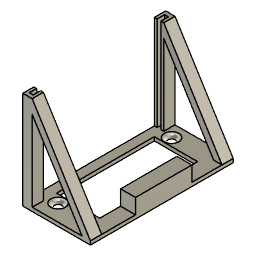
Light Mount Bracket (Autodesk Fusion 360 design; units mm, degrees)
Autodesk Fusion 360 part; units mm, degrees
sketch "Sketch1" plane through (0, 0, 0) normal (0, 0, 1) x (1, 0, 0)
  line L0 (-5, 11) -> (31, 11)
  line L1 (31, 11) -> (31, -65)
  line L2 (31, -65) -> (-5, -65)
  line L3 (-5, -65) -> (-5, 11)
  line L4 (0, 0) -> (23, 0)
  line L5 (23, 0) -> (23, -52)
  line L6 (23, -52) -> (0, -52)
  line L7 (0, -52) -> (0, 0)
  circle A0 centre (5, -56.1622) radius 1.9
  circle A1 centre (5, 4.1628) radius 1.9
  dimension "d1" = 76
  dimension "d2" = 36
  dimension "d3" = 23
  dimension "d4" = 3.8
  dimension "d5" = 60.325
  dimension "d8" = 10
  dimension "d19" = 5
  dimension "d20" = 10
  dimension "d21" = 4.1622
  dimension "d22" = 13
  constraint horizontal L0
  constraint vertical L1
  constraint horizontal L2
  constraint vertical L3
  constraint horizontal L4
  constraint vertical L5
  constraint horizontal L6
  constraint vertical L7
  constraint coincident L4.start L7.end
  constraint equal A0 A1
  measures "d1" distance of L0.start L2.end
  measures "d2" distance of L0.start L0.end
  measures "d3" distance of L4.start L4.end
  measures "d4" diameter of A0
  measures "d5" distance of A0.centre A1.centre
  measures "d8" distance of L3 A0.centre
  measures "d19" distance of L3 L7
  measures "d20" distance of L3 A1.centre
  measures "d21" distance of L6 A0.centre
  measures "d22" distance of L2 L6
extrude "Extrude1" add sketch "Sketch1" along normal blind 2
fillet "Fillet1" radius 2 2 edges at (3.2286, 4.8499, 2) (3.2286, -55.4751, 2)
sketch "Sketch2" plane through (0, 0, 2) normal (0, 0, 1) x (-1, 0, 0)
  circle A0 centre (-5, -4.1628) radius 3.9
  line L0 (-23, 52) -> (0, 52)
  line L1 (0, 52) -> (0, 0)
  line L2 (0, 0) -> (-23, 0)
  line L3 (-23, 0) -> (-23, 52)
  line L4 (5, 65) -> (-31, 65)
  line L5 (-31, 65) -> (-31, -11)
  line L6 (-31, -11) -> (5, -11)
  line L7 (5, -11) -> (5, 65)
  circle A1 centre (-5, 56.1622) radius 3.9
  line L8 (-23, 11) -> (-31, 11)
  line L9 (-31, 11) -> (-31, 41)
  line L10 (-31, 41) -> (-23, 41)
  line L11 (-23, 41) -> (-23, 11)
  dimension "d17" = 30
  dimension "d18" = 22
  constraint horizontal L8
  constraint vertical L9
  constraint horizontal L10
  constraint vertical L11
  constraint coincident L5 L9.end
  constraint collinear L3 L11
  measures "d17" distance of L8 L10
  measures "d18" distance of L6 L8
extrude "Extrude2" add sketch "Sketch2" along normal blind 8 contours L3 L5 L8 L9 L10 L11
sketch "Sketch3" plane through (23, 0, 0) normal (-1, 0, 0) x (0, -1, 0)
  line L0 (0, 0) -> (52, 0)
  line L1 (52, 0) -> (52, 2)
  line L2 (0, 2) -> (0, 0)
  circle A0 centre (26, 7.5) radius 0.625
  line L3 (52, 2) -> (41, 2)
  line L4 (11, 2) -> (0, 2)
  line L5 (41, 2) -> (41, 10)
  line L6 (41, 10) -> (11, 10)
  line L7 (11, 10) -> (11, 2)
  dimension "d16" = 1.25
  dimension "d37" = 2.5
  dimension "d38" = 15
  measures "d16" diameter of A0
  measures "d37" distance of A0.centre L6
  measures "d38" distance of A0.centre L7
extrude "Extrude3" cut sketch "Sketch3" against normal blind 5 contours A0
sketch "Sketch4" plane through (0, 0, 2) normal (0, 0, 1) x (-1, 0, 0)
  line L0 (-23, 11) -> (-31, 11)
  line L1 (-31, 11) -> (-31, -11)
  line L2 (-31, -11) -> (5, -11)
  line L3 (5, -11) -> (5, 65)
  line L4 (5, 65) -> (-31, 65)
  line L5 (-31, 65) -> (-31, 41)
  line L6 (-31, 41) -> (-23, 41)
  line L7 (-23, 41) -> (-23, 52)
  line L8 (-23, 52) -> (0, 52)
  line L9 (0, 52) -> (0, 0)
  line L10 (0, 0) -> (-23, 0)
  line L11 (-23, 0) -> (-23, 11)
  circle A0 centre (-5, -4.1628) radius 3.9
  circle A1 centre (-5, 56.1622) radius 3.9
  line L12 (5, -11) -> (-0.033, -11)
  line L13 (-0.033, -11) -> (-0.033, 65)
  line L14 (-0.033, 65) -> (5, 65)
  line L15 (5, 65) -> (5, -11)
  constraint horizontal L12
  constraint vertical L13
  constraint horizontal L14
  constraint vertical L15
  constraint coincident L4 L13.end
  constraint coincident L2.end L3.start
extrude "Extrude4" add sketch "Sketch4" along normal blind 50 contours L8 L9 L10 L13 | L2 L3 L4 L8 L9 L10 L12 L13 L14 L15
sketch "Sketch5" plane through (0, 0, 52) normal (0, 0, 1) x (-1, 0, 0)
  line L0 (5, 65) -> (-0.033, 65)
  line L1 (-0.033, 65) -> (-0.033, -11)
  line L2 (-0.033, -11) -> (5, -11)
  line L3 (5, -11) -> (5, 65)
  line L4 (3.467, -9) -> (1.467, -9)
  line L5 (1.467, -9) -> (1.467, 63)
  line L6 (1.467, 63) -> (3.467, 63)
  line L7 (3.467, 63) -> (3.467, -9)
  line L8 (5, -5) -> (-0.033, -5)
  line L9 (-0.033, -5) -> (-0.033, 59)
  line L10 (-0.033, 59) -> (5, 59)
  line L11 (5, 59) -> (5, -5)
  dimension "d25" = 2
  dimension "d26" = 72
  dimension "d27" = 2
  dimension "d28" = 1.5
  dimension "d29" = 64
  dimension "d30" = 4
  constraint horizontal L4
  constraint vertical L5
  constraint horizontal L6
  constraint vertical L7
  constraint horizontal L8
  constraint vertical L9
  constraint horizontal L10
  constraint vertical L11
  constraint coincident L1 L9.end
  constraint coincident L3 L8.start
  measures "d25" distance of L4.start L4.end
  measures "d26" distance of L4.start L6.end
  measures "d27" distance of L2 L4
  measures "d28" distance of L1 L5
  measures "d29" distance of L8 L10
  measures "d30" distance of L4 L8
extrude "Extrude5" cut sketch "Sketch5" against normal blind 50 contours L3 L7 L8 L10 L11 | L1 L5 L8 L9 L10 | L5 L6 L7 L10 | L5 L7 L8 L10 | L4 L5 L7 L8
sketch "Sketch6" plane through (0, -65, 0) normal (0, -1, 0) x (1, 0, 0)
  line L0 (-5, 0) -> (31, 0)
  line L1 (31, 0) -> (31, 2)
  line L2 (31, 2) -> (0.033, 2)
  line L3 (0.033, 2) -> (0.033, 52)
  line L4 (0.033, 52) -> (-5, 52)
  line L5 (-5, 52) -> (-5, 0)
  line L6 (0.033, 52) -> (31, 2)
  line L7 (31, 2) -> (27.7819, 0.0069)
  line L8 (27.7819, 0.0069) -> (-3.185, 50.0069)
  line L9 (-3.185, 50.0069) -> (0.033, 52)
  constraint perpendicular L6 L7
  constraint parallel L6 L8
  constraint parallel L7 L9
  constraint coincident L1.end L2.start
  constraint coincident L3.end L4.start
extrude "Extrude6" add sketch "Sketch6" against normal blind 6 contours L2 L3 L6 L8
sketch "Sketch7" plane through (0, 11, 0) normal (0, 1, 0) x (-1, 0, 0)
  line L0 (-31, 0) -> (5, 0)
  line L1 (5, 0) -> (5, 52)
  line L2 (5, 52) -> (-0.033, 52)
  line L3 (-0.033, 52) -> (-0.033, 2)
  line L4 (-0.033, 2) -> (-31, 2)
  line L5 (-31, 2) -> (-31, 0)
  line L6 (-0.033, 52) -> (-31, 2)
  line L7 (-31, 2) -> (-27.7819, 0.0069)
  line L8 (-27.7819, 0.0069) -> (3.185, 50.0069)
  line L9 (3.185, 50.0069) -> (-0.033, 52)
  constraint perpendicular L6 L7
  constraint parallel L6 L8
  constraint parallel L7 L9
  constraint coincident L4.end L5.start
  constraint coincident L2.end L3.start
extrude "Extrude7" add sketch "Sketch7" against normal blind 6 contours L3 L4 L6 L8
equation "d20 = d8"
